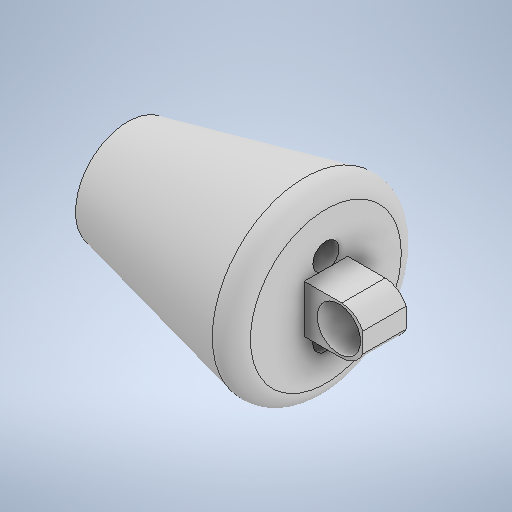
# Autodesk Inventor part: thumb 6th part(model 2)
Saved by Autodesk Inventor 2025 (Build 290162000, 162)
## iProperties
Created: 2025-11-10
Part Number: thumb 6th part(model 2)
Material: Generic
Document SubType Name: Modeling
Designer: abdul
Density: 1 g/cm^3
Appearance: Default
Author: abdul
Autodesk Inventor part; units mm, degrees
ref_plane "YZ Plane" through (0, 0, 0) normal (1, 0, 0) x (0, 1, 0)
ref_plane "XZ Plane" through (0, 0, 0) normal (0, 1, 0) x (-1, 0, 0)
ref_plane "XY Plane" through (0, 0, 0) normal (0, 0, 1) x (1, 0, 0)
sketch "Sketch1" plane through (0, 0, 0) normal (0, 1, 0) x (-1, 0, 0)
  line L0 (0, 0) -> (0, -10)
  line L1 (17.5988, 0) -> (17.5988, -6)
  line L2 (17.5988, -6) -> (0, -10)
  line L3 (17.5988, 0) -> (0, 0)
  dimension "d0" = 10
  dimension "d2" = 6
  dimension "d3" = 77.195
  dimension "d4" = 17.5988
  constraints: 8 end point, 2 vertical
  measures "d0" distance of L0.start L0.end
  measures "d2" distance of L1.start L1.end
  measures "d3" angle of L2 L1
  measures "d4" distance between parallel lines of L0 L1
revolve "Revolution1" add sketch "Sketch1" angle 360 about axis through (-17.5988, 0, 0) along (1, 0, 0)
sketch "Sketch2" plane through (0, 0, 0) normal (0, 0, 1) x (1, 0, 0)
  point P0 (0, 0)
sketch "Sketch3" plane through (0, 0, 0) normal (1, 0, 0) x (0, 0, -1)
  line L0 (-2.5, 2.75) -> (2.5, 2.75)
  line L1 (2.5, 2.75) -> (2.5, -2.75)
  line L2 (2.5, -2.75) -> (-2.5, -2.75)
  line L3 (-2.5, -2.75) -> (-2.5, 2.75)
  line L4 (-2.5, 2.75) -> (2.5, -2.75) construction
  line L5 (2.5, 2.75) -> (-2.5, -2.75) construction
  point P0 (0, 0)
  dimension "d6" = 5.5
  dimension "d7" = 5
  constraints: 12 end point, 2 midpoint, 2 parallel, 1 horizontal, 1 perpendicular
  measures "d6" distance of L0.end L1.end
  measures "d7" distance of L1.end L2.end
extrude "Extrusion1" add sketch "Sketch3" along normal blind 6.75
sketch "Sketch4" plane through (0, -2.75, -2.5) normal (0, 0, -1) x (-1, 0, 0)
  circle A0 centre (-4, 2.75) radius 2.5
  line L0 (0, 5.5) -> (0, 0) projected
  point P0 (0, 2.75)
  dimension "d10" = 5
  dimension "d11" = 4
  constraints: 1 centre point
  measures "d10" diameter of A0
  measures "d11" distance from line of L0 A0.centre
extrude "Extrusion2" cut sketch "Sketch4" against normal blind 7
sketch "Sketch5" plane through (0, -2.75, -2.5) normal (0, 0, -1) x (-1, 0, 0)
  line L0 (0, 5.5) -> (-6.75, 5.5) projected
  line L1 (0, 0) -> (-6.75, 0) projected
  line L2 (-4.3613, 0) -> (-6.75, 0)
  line L3 (-6.75, 5.5) -> (-6.75, 0) projected
  line L4 (-6.75, 5.5) -> (-4.3345, 5.5)
  arc A0 (-4.3345, 5.5) -> (-4.3613, 0) centre (-4.2482, 2.7495) ccw
  point P0 (0, 2.75)
  point P1 (-6.75, 3.8956)
  point P2 (-6.75, 1.6035)
  constraints: 4 end point, 2 point on circle, 2 point on line, 1 centre point, 1 collinear
extrude "Extrusion3" cut sketch "Sketch5" against normal blind 7 contours A0 L3 L0 | A0 L1 L3
fillet "Fillet1" radius 2 1 edges at (0, 0, 10)
sketch "Sketch6" plane through (0, 0, 0) normal (1, 0, 0) x (0, 0, -1)
  circle A0 centre (0, -4) radius 1.5
  line L0 (0, 0) -> (-4.6959, 0)
  circle A1 centre (0, 4) radius 1.5
  dimension "d17" = 3
  dimension "d19" = 4
  constraints: 2 centre point, 2 end point, 1 horizontal, 1 symmetric about line, 1 other
  measures "d17" diameter of A0
  measures "d19" distance of L0.start A0.centre
extrude "Extrusion4" cut sketch "Sketch6" against normal through all
move faces "Move1" translate (-5.25, 0, 0) faces at (-17.5988, 0, -2.5681) (-5.8112, -2.0771, -8.427)
body "Solid1"
